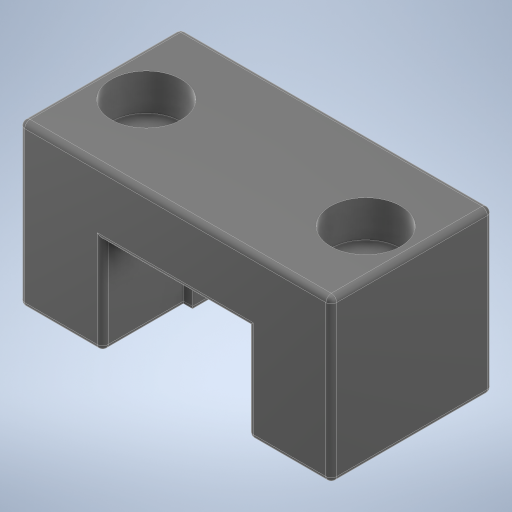
# Autodesk Inventor part: connector_securing_V1
Saved by Autodesk Inventor 2023 (Build 270158000, 158)
## iProperties
Created: 2023-10-05
Part Number: connector_securing_V1
Material: ABS-Kunststoff
Document SubType Name: Modeling
Designer: Mathi
Density: 1.06 g/cm^3
Appearance: Glatt - Weiß
Author: Mathi
Autodesk Inventor part; units mm, degrees
ref_plane "YZ Plane" through (0, 0, 0) normal (1, 0, 0) x (0, 1, 0)
ref_plane "XZ Plane" through (0, 0, 0) normal (0, 1, 0) x (-1, 0, 0)
ref_plane "XY Plane" through (0, 0, 0) normal (0, 0, 1) x (1, 0, 0)
sketch "Skizze1" plane through (0, 0, 0) normal (0, 0, 1) x (1, 0, 0)
  line L0 (-14.5, 0) -> (14.5, 0)
  line L1 (14.5, 0) -> (14.5, -15)
  line L2 (-14.5, -15) -> (-14.5, 0)
  line L3 (-5.9, -15) -> (-5.9, -6.6)
  line L4 (-5.9, -6.6) -> (5.9, -6.6)
  line L5 (5.9, -6.6) -> (5.9, -15)
  line L6 (14.5, -15) -> (5.9, -15)
  line L7 (-5.9, -15) -> (-14.5, -15)
  line L8 (0, 0) -> (0, -6.6)
  line L9 (-10.2, -15) -> (-10.2, 0)
  line L10 (10.2, -15) -> (10.2, 0)
  dimension "d0" = 11.8
  dimension "d1" = 8.4
  dimension "d2" = 29
  dimension "d3" = 15
  constraints: 22 end point, 5 perpendicular, 4 midpoint, 3 parallel, 3 point on line, 2 horizontal, 2 vertical
  measures "d0" distance between parallel lines of L5 L3
  measures "d1" distance between parallel lines of L4 L6
  measures "d2" distance between parallel lines of L1 L2
  measures "d3" distance of L2.start L0.start
extrude "Extrusion1" add sketch "Skizze1" along normal mid plane 15
sketch "Skizze2" plane through (0, 0, 0) normal (0, 0, 1) x (1, 0, 0)
  line L0 (5.9, -15) -> (14.5, -15) projected
  line L1 (6.75, -15) -> (-6.75, -15)
  line L2 (-6.75, -15) -> (-6.75, -6)
  line L3 (-6.75, -6) -> (6.75, -6)
  line L4 (6.75, -6) -> (6.75, -15)
  line L5 (0, -18) -> (0, 3) projected
  point P0 (0, 0)
  point P1 (0, -6)
  dimension "d6" = 13.5
  dimension "d7" = 9
  constraints: 8 end point, 2 parallel, 2 point on line, 1 horizontal, 1 midpoint, 1 perpendicular
  measures "d6" distance between parallel lines of L4 L2
  measures "d7" distance between parallel lines of L0 L3
extrude "Extrusion2" cut sketch "Skizze2" along normal through all
sketch "Skizze3" plane through (-14.5, 0, 7.5) normal (0, 1, 0) x (1, 0, 0)
  point P0 (14.5, 7.5)
  point P1 (4.3, 7.5)
  point P2 (24.7, 7.5)
hole "Bohrung1" at (-10.2, 0, 0) at (10.2, 0, 0) direction (0, -1, 0) diameter 3 end through all counterbore diameter 6.5 counterbore depth 3.4 clearance for "Inbusschraube DIN EN ISO 4762" size "M3" standard "DIN"
fillet "Rundung1" radius 0.5 26 edges at (0, 0, 7.5) (14.5, 0, 0) (0, 0, -7.5) (-14.5, 0, 0) (-6.75, -10.5, 7.5) (0, -6, 7.5) (-10.625, -15, 7.5) (-14.5, -7.5, 7.5) (6.75, -10.5, 7.5) (10.625, -15, 7.5) (14.5, -7.5, 7.5) (14.5, -7.5, -7.5) (14.5, -15, 0) (5.9, -10.8, -7.5) (0, -6.6, -7.5) (-5.9, -10.8, -7.5) (-14.5, -7.5, -7.5) (-10.2, -15, -7.5) (-5.9, -15, -3.75) (-6.75, -15, 3.75) (-14.5, -15, 0) (-6.325, -15, 0) (6.325, -15, 0) (6.75, -15, 3.75) (5.9, -15, -3.75) (10.2, -15, -7.5)
